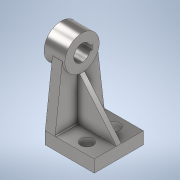
# Autodesk Inventor part: Soporte_Tensor
Saved by Autodesk Inventor 2021 (Build 250183000, 183)
## iProperties
Created: 2020-12-29
Part Number: Soporte_Tensor
Material: Iron, Malleable
Document SubType Name: Modeling
Designer: mauro
Density: 7.15 g/cm^3
Appearance: Semi-Polished
Author: mauro
Autodesk Inventor part; units mm, degrees
ref_plane "YZ Plane" through (0, 0, 0) normal (1, 0, 0) x (0, 1, 0)
ref_plane "XZ Plane" through (0, 0, 0) normal (0, 1, 0) x (-1, 0, 0)
ref_plane "XY Plane" through (0, 0, 0) normal (0, 0, 1) x (1, 0, 0)
sketch "Boceto2" plane through (0, 0, 0) normal (0, 1, 0) x (-1, 0, 0)
  line L0 (0, 0) -> (0, 40) construction
  line L1 (0, 40) -> (-47, 40)
  line L2 (-47, 40) -> (-47, 0)
  line L3 (-47, 0) -> (-47, -40)
  line L4 (-47, 0) -> (-17, 0) construction
  line L5 (-17, 0) -> (-17, -22) construction
  circle A0 centre (-17, -22) radius 10
  line L6 (-17, 0) -> (-17, 22) construction
  circle A1 centre (-17, 22) radius 10
  line L7 (-47, 0) -> (-47, -4) construction
  line L8 (-47, -4) -> (13, -4)
  line L9 (-47, 0) -> (-47, 4) construction
  line L10 (17, 40) -> (17, 28)
  line L11 (17, -28) -> (17, -40)
  line L12 (33, -40) -> (33, -28)
  line L13 (-47, -40) -> (0, -40)
  line L14 (0, -40) -> (17, -40)
  line L15 (33, -40) -> (17, -40)
  line L16 (0, 40) -> (17, 40)
  line L17 (33, 28) -> (33, 40)
  line L18 (47, 40) -> (33, 40) construction
  line L19 (33, 40) -> (17, 40)
  line L20 (13, -40) -> (47, -40) construction
  line L21 (33, 28) -> (33, -28)
  line L22 (17, 28) -> (17, -28)
  line L23 (-47, 4) -> (17, 4)
  line L24 (13, -4) -> (17, -4)
  line L25 (47, -40) -> (47, 40) construction
  line L26 (-47, 0) -> (17, 0)
  dimension "d2" = 40
  dimension "d4" = 47
  dimension "d5" = 40
  dimension "d10" = 30
  dimension "d11" = 22
  dimension "d12" = 20
  dimension "d16" = 4
  dimension "d17" = 4
  dimension "d41" = 16
  dimension "d44" = 34
  constraints: 54 end point, 7 horizontal, 6 point on line, 4 collinear, 3 perpendicular, 3 vertical, 2 centre point, 2 coincident, 2 symmetric about line, 1 midpoint, 1 other
  measures "d2" distance of L0.start L0.end
  measures "d4" distance of L0.end L1.end
  measures "d5" distance of L2.end L3.end
  measures "d10" distance of L2.end L4.end
  measures "d11" distance of L4.end L5.end
  measures "d12" diameter of A0
  measures "d16" distance of L2.end L7.end
  measures "d17" distance of L2.end L9.end
  measures "d41" distance of L12.start L11.end
  measures "d44" distance of L20.start L20.end
extrude "Extrusión5" add sketch "Boceto2" along normal blind 20 contours L16 L10 L22 L23 L2 L1 | L8 L24 L22 L11 L14 L13 L3
extrude "Extrusión8" add sketch "Boceto2" along normal blind 120 contours L19 L17 L21 L12 L15 L11 L22 L10
sketch "Boceto12" plane through (-33, 0, -40) normal (-1, 0, 0) x (0, 0, 1)
  line L0 (0, 20) -> (0, 120) projected
  line L1 (0, 0) -> (0, 20)
  line L2 (80, 0) -> (80, 20) projected
  line L3 (0, 20) -> (80, 20)
  line L4 (80, 20) -> (80, 0)
  line L5 (80, 0) -> (0, 0)
  line L6 (40, 0) -> (40, 120) construction
  circle A0 centre (40, 120) radius 28
  arc A1 (27.1062, 116) -> (27.1062, 124) centre (40, 120) ccw
  line L7 (12.1931, 123.2828) -> (0, 20)
  line L8 (67.8069, 123.2828) -> (80, 20)
  line L9 (0, 120) -> (80, 120) projected
  line L10 (53.5, 120) -> (23.2, 120) construction
  line L11 (23.2, 120) -> (23.2, 124)
  line L12 (23.2, 124) -> (27.1062, 124)
  line L13 (23.2, 120) -> (23.2, 116)
  line L14 (23.2, 116) -> (27.1062, 116)
  line L15 (80, 120) -> (0, 120) projected
  line L16 (80, 120) -> (80, 22.7295)
  line L17 (80, 20) -> (80, 120) projected
  point P0 (68, 120)
  point P1 (68.1944, 120)
  point P2 (11.8056, 120)
  dimension "d68" = 56
  dimension "d69" = 27
  dimension "d70" = 30.3
  constraints: 26 end point, 5 point on circle, 4 perpendicular, 3 point on line, 3 vertical, 2 centre point, 2 coincident, 2 tangent, 1 collinear, 1 horizontal
  measures "d68" diameter of A0
  measures "d69" diameter of A1
  measures "d70" distance of L10.start L10.end
extrude "Extrusión9" add sketch "Boceto12" along normal blind 14 and the other way blind 20 contours A0 L9 A1 L12 L11 | L9 L13 L14 A1 A0
extrude "Extrusión10" cut sketch "Boceto12" against normal blind 30 contours L0 L9 L7 | L8 L9 L16 L17 | L9 A1 L14 L13
extrude "Extrusión13" add sketch "Boceto2" along normal blind 92 contours L23 L22 L26 L2 | L26 L22 L24 L8 L3
sketch "Boceto15" plane through (-17, 20, 4) normal (0, 0, 1) x (1, 0, 0)
  arc A0 (-16, 70) -> (-18, 72) centre (-18, 70) ccw
  arc A1 (0, 2) -> (2, 0) centre (2, 2) ccw
  arc A2 (2, 72) -> (0, 70) centre (2, 70) ccw
  line L0 (0, 72) -> (64, 72) projected
  line L1 (0, 100) -> (0, 0) projected
  line L2 (-16, 0) -> (-16, 100) projected
  line L3 (-30, 128) -> (-30, 72) projected
  line L4 (-30, 72) -> (-16, 72)
  line L5 (0, 0) -> (64, 0) projected
  line L6 (64, 72) -> (0, 72) projected
  line L7 (0, 72) -> (4, 72)
  line L8 (4, 72) -> (64, 0)
  line L9 (4, 72) -> (64, 72)
  line L10 (64, 72) -> (64, 0)
  point P0 (17, -20)
  point P1 (4, 72)
  dimension "d90" = 4
  dimension "d92" = 4
  dimension "d93" = 4
  dimension "d94" = 4
  constraints: 10 end point, 8 point on line, 6 point on circle, 6 tangent, 3 centre point, 1 collinear, 1 perpendicular
  measures "d90" diameter of A0
  measures "d92" diameter of A1
  measures "d93" diameter of A2
  measures "d94" distance of L0.start L7.end
extrude "Extrusión14" cut sketch "Boceto15" against normal blind 20 contours L8 L0 L10
extrude "Extrusión15" add sketch "Boceto15" along normal blind 36 and the other way blind 44 contours A1 L5 L1
